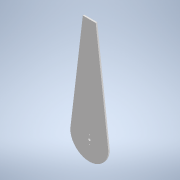
# Autodesk Inventor part: ухо
Saved by Autodesk Inventor 2021.1 (Build 251245010, 245A)
## iProperties
Created: 2023-01-27
Part Number: ухо
Material: Типовые
Document SubType Name: Modeling
Designer: zmoze
Density: 1 g/cm^3
Appearance: По умолчанию
Author: zmoze
Autodesk Inventor part; units mm, degrees
ref_plane "YZ Plane" through (0, 0, 0) normal (1, 0, 0) x (0, 1, 0)
ref_plane "XZ Plane" through (0, 0, 0) normal (0, 1, 0) x (-1, 0, 0)
ref_plane "XY Plane" through (0, 0, 0) normal (0, 0, 1) x (1, 0, 0)
sketch "Эскиз1" plane through (0, 0, 0) normal (0, 0, 1) x (1, 0, 0)
  circle A0 centre (0, 0) radius 40
  line L0 (-40, 0) -> (-13.6038, 219.402)
  line L1 (-13.6038, 219.402) -> (13.6038, 219.402)
  line L2 (13.6038, 219.402) -> (40, 0)
  line L3 (0, 0) -> (0, 40) construction
  line L4 (0, 0) -> (40, 0) construction
  point P0 (0, 219.402)
  dimension "d0" = 80
  constraints: 10 end point, 3 point on circle, 2 horizontal, 1 centre point, 1 coincident, 1 equal length, 1 midpoint, 1 point on line, 1 vertical
  measures "d0" diameter of A0
extrude "Выдавливание1" add sketch "Эскиз1" along normal blind 3 contours L0 A0 L2 | L0 L1 L2 A0
sketch "Эскиз2" plane through (0, 0, 3) normal (0, 0, 1) x (1, 0, 0)
  arc A0 (3, 2.25) -> (-3, 2.25) centre (0, 0) ccw construction
  line L0 (-1.9929, 14.1684) -> (-3, 2.25) construction
  arc A1 (1.9929, 14.1684) -> (-1.9929, 14.1684) centre (0, 14) ccw construction
  line L1 (3, 2.25) -> (1.9929, 14.1684) construction
  circle A2 centre (0, 13) radius 0.5 construction
  circle A3 centre (0, 11) radius 0.5 construction
  circle A4 centre (0, 9) radius 0.5 construction
  circle A5 centre (0, 7) radius 0.5 construction
  circle A6 centre (0, 5) radius 0.5 construction
  circle A7 centre (0, 15) radius 0.5 construction
  arc A8 (-1.9929, -14.1684) -> (1.9929, -14.1684) centre (0, -14) ccw construction
  line L2 (-3, -2.25) -> (-1.9929, -14.1684) construction
  arc A9 (-3, -2.25) -> (3, -2.25) centre (0, 0) ccw construction
  line L3 (1.9929, -14.1684) -> (3, -2.25) construction
  circle A10 centre (0, -5) radius 0.5 construction
  circle A11 centre (0, -7) radius 0.5 construction
  circle A12 centre (0, -9) radius 0.5 construction
  circle A13 centre (0, -11) radius 0.5 construction
  circle A14 centre (0, -13) radius 0.5 construction
  circle A15 centre (0, -15) radius 0.5 construction
  circle A16 centre (0, 0) radius 2.3 projected
  circle A17 centre (0, 9) radius 1
  circle A18 centre (0, -9) radius 1
  point P0 (0, 0)
  dimension "d3" = 2
  dimension "d4" = 2
  constraints: 2 centre point, 2 coincident
  measures "d3" diameter of A17
  measures "d4" diameter of A18
extrude "Выдавливание2" cut sketch "Эскиз2" against normal blind 10
